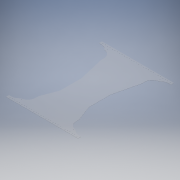
# Autodesk Inventor part: Belly Pan
Saved by Autodesk Inventor 2019.4 (Build 234330000, 330)
## iProperties
Created: 2019-12-14
Part Number: Belly Pan
Material: Polycarbonate, Clear
Document SubType Name: Modeling
Designer: Mark
Density: 1.2 g/cm^3
Appearance: Polycarbonate - Clear
Mass: 741.672 g
Surface Area: 6247.34 cm^2
Volume: 618.06 cm^3
Author: Mark
Autodesk Inventor part; units mm, degrees
ref_plane "YZ Plane" through (0, 0, 0) normal (1, 0, 0) x (0, 1, 0)
ref_plane "XZ Plane" through (0, 0, 0) normal (0, 1, 0) x (-1, 0, 0)
ref_plane "XY Plane" through (0, 0, 0) normal (0, 0, 1) x (1, 0, 0)
sketch "Sketch1" plane through (0, 0, 0) normal (0, 1, 0) x (-1, 0, 0)
  line L0 (-230, 400) -> (230, 400)
  line L1 (230, 400) -> (230, -400)
  line L2 (230, -400) -> (-230, -400)
  line L3 (-230, -400) -> (-230, 400)
  line L4 (-230, 400) -> (230, -400) construction
  line L5 (230, 400) -> (-230, -400) construction
  line L6 (230, 400) -> (300, 400)
  line L7 (300, 400) -> (300, 375)
  line L8 (300, 375) -> (230, 375)
  line L9 (230, 375) -> (230, 400)
  line L10 (230, -400) -> (300, -400)
  line L11 (300, -400) -> (300, -375)
  line L12 (300, -375) -> (230, -375)
  line L13 (230, -375) -> (230, -400)
  line L14 (-230, -400) -> (-300, -400)
  line L15 (-300, -400) -> (-300, -375)
  line L16 (-300, -375) -> (-230, -375)
  line L17 (-230, -375) -> (-230, -400)
  line L18 (-230, 400) -> (-300, 400)
  line L19 (-300, 400) -> (-300, 375)
  line L20 (-300, 375) -> (-230, 375)
  line L21 (-230, 375) -> (-230, 400)
  line L22 (-230, 217.5) -> (-300, 217.5)
  line L23 (-300, 217.5) -> (-300, 192.5)
  line L24 (-300, 192.5) -> (-230, 192.5)
  line L25 (-230, 192.5) -> (-230, 217.5)
  line L26 (230, 217.5) -> (300, 217.5)
  line L27 (300, 217.5) -> (300, 192.5)
  line L28 (300, 192.5) -> (230, 192.5)
  line L29 (230, 192.5) -> (230, 217.5)
  line L30 (-230, -227.5) -> (-300, -227.5)
  line L31 (-300, -227.5) -> (-300, -202.5)
  line L32 (-300, -202.5) -> (-230, -202.5)
  line L33 (-230, -202.5) -> (-230, -227.5)
  line L34 (-230, -87.5) -> (-300, -87.5)
  line L35 (-300, -87.5) -> (-300, -62.5)
  line L36 (-300, -62.5) -> (-230, -62.5)
  line L37 (-230, -62.5) -> (-230, -87.5)
  line L38 (0, 0) -> (0, -50)
  line L39 (0, 0) -> (50, 0) construction
  line L40 (230, -227.5) -> (300, -227.5)
  line L41 (300, -227.5) -> (300, -202.5)
  line L42 (300, -202.5) -> (230, -202.5)
  line L43 (230, -202.5) -> (230, -227.5)
  line L44 (230, -87.5) -> (300, -87.5)
  line L45 (300, -87.5) -> (300, -62.5)
  line L46 (300, -62.5) -> (230, -62.5)
  line L47 (230, -62.5) -> (230, -87.5)
  dimension "d0" = 460
  dimension "d1" = 800
  dimension "d26" = 70
  dimension "d27" = 25
  dimension "d28" = 70
  dimension "d29" = 25
  dimension "d30" = 70
  dimension "d31" = 25
  dimension "d32" = 70
  dimension "d33" = 70
  dimension "d34" = 25
  dimension "d35" = 182.5
  dimension "d36" = 70
  dimension "d37" = 25
  dimension "d38" = 182.5
  dimension "d39" = 70
  dimension "d40" = 25
  dimension "d41" = 172.5
  dimension "d42" = 70
  dimension "d43" = 25
  dimension "d44" = 312.5
  dimension "d45" = 50
  dimension "d46" = 90
  constraints: 96 end point, 18 parallel, 10 horizontal, 10 perpendicular, 8 symmetric about line, 5 point on line, 2 midpoint, 1 vertical
  measures "d0" distance of L1.end L2.end
  measures "d1" distance of L0.end L1.end
  measures "d26" distance of L7.end L8.end
  measures "d27" distance of L6.end L7.end
  measures "d28" distance of L12.end L11.end
  measures "d29" distance of L11.end L10.end
  measures "d30" distance of L15.end L16.end
  measures "d31" distance of L14.end L15.end
  measures "d32" distance of L20.end L19.end
  measures "d33" distance of L24.end L23.end
  measures "d34" distance of L23.end L22.end
  measures "d35" distance between parallel lines of L18 L22
  measures "d36" distance of L27.end L28.end
  measures "d37" distance of L26.end L27.end
  measures "d38" distance between parallel lines of L26 L6
  measures "d39" distance of L31.end L32.end
  measures "d40" distance of L30.end L31.end
  measures "d41" distance between parallel lines of L2 L30
  measures "d42" distance of L35.end L36.end
  measures "d43" distance of L34.end L35.end
  measures "d44" distance between parallel lines of L2 L34
  measures "d45" distance of L38.start L38.end
  measures "d46" angle of L38 L39
extrude "Extrusion1" add sketch "Sketch1" along normal blind 2 contours L0 L1 L2 L3 | L3 L20 L19 L18 | L6 L7 L8 L1 | L3 L14 L15 L16 | L12 L11 L10 L1
sketch "Sketch2" plane through (0, 2, 0) normal (0, 1, 0) x (1, 0, 0)
  line L0 (-230, 375) -> (-230, -375) projected
  line L1 (-230, -130) -> (-120, -130)
  line L2 (-120, -130) -> (-120, 50)
  line L3 (-120, 50) -> (-230, 50)
  line L4 (-230, 50) -> (-230, -130)
  line L5 (300, 400) -> (-300, 400) projected
  line L6 (230, -130) -> (120, -130)
  line L7 (120, -130) -> (120, 50)
  line L8 (120, 50) -> (230, 50)
  line L9 (230, 50) -> (230, -130)
  line L10 (230, -375) -> (230, 375) projected
  line L11 (-230, -40) -> (230, -40) construction
  line L12 (-230, -40) -> (230, -40) construction
  line L13 (-230, -347.5) -> (-170, -347.5)
  line L14 (-170, -347.5) -> (-170, -262.5)
  line L15 (-170, -262.5) -> (-230, -262.5)
  line L16 (-230, -262.5) -> (-230, -347.5)
  line L17 (-300, -400) -> (300, -400) projected
  line L18 (0, -400) -> (0, -300) construction
  line L19 (0, -400) -> (100, -400) construction
  line L20 (230, -347.5) -> (170, -347.5)
  line L21 (170, -347.5) -> (170, -262.5)
  line L22 (170, -262.5) -> (230, -262.5)
  line L23 (230, -262.5) -> (230, -347.5)
  line L24 (-230, 182.5) -> (-230, 267.5)
  line L25 (-230, 347.5) -> (-170, 347.5)
  line L26 (-170, 347.5) -> (-170, 262.5)
  line L27 (-170, 262.5) -> (-230, 262.5)
  line L28 (-230, 262.5) -> (-230, 347.5)
  line L29 (230, 347.5) -> (170, 347.5)
  line L30 (170, 347.5) -> (170, 262.5)
  line L31 (170, 262.5) -> (230, 262.5)
  line L32 (230, 262.5) -> (230, 347.5)
  line L33 (120, 50) -> (170, 262.5)
  line L34 (120, -130) -> (170, -262.5)
  line L35 (-170, -262.5) -> (-120, -130)
  line L36 (-120, -130) -> (-230, -130)
  line L37 (-230, -262.5) -> (-230, -130)
  line L38 (-230, -262.5) -> (-170, -262.5)
  line L39 (-120, 50) -> (-230, 50)
  line L40 (-230, 50) -> (-230, 262.5)
  line L41 (-230, 262.5) -> (-170, 262.5)
  line L42 (-170, 262.5) -> (-120, 50)
  line L43 (-170, -262.5) -> (-230, -262.5)
  line L44 (-230, -262.5) -> (-230, -130)
  line L45 (-230, -130) -> (-120, -130)
  line L46 (-120, -130) -> (-170, -262.5)
  line L47 (-230, 50) -> (-230, 262.5)
  line L48 (-230, 262.5) -> (-170, 262.5)
  line L49 (-170, 262.5) -> (-120, 50)
  line L50 (-120, 50) -> (-230, 50)
  line L51 (120, 50) -> (230, 50)
  line L52 (230, 262.5) -> (230, 50)
  line L53 (120, 50) -> (170, 262.5)
  line L54 (170, 262.5) -> (230, 262.5)
  line L55 (170, -262.5) -> (120, -130)
  line L56 (120, -130) -> (230, -130)
  line L57 (230, -262.5) -> (170, -262.5)
  line L58 (230, -262.5) -> (230, -130)
  point P0 (0, 0)
  point P1 (-230, 400)
  point P2 (-230, -400)
  point P3 (230, 400)
  point P4 (230, -400)
  point P5 (-230, -192.5)
  point P6 (230, -217.5)
  point P7 (-230, 87.5)
  dimension "d4" = 110
  dimension "d5" = 180
  dimension "d6" = 350
  dimension "d7" = 110
  dimension "d8" = 180
  dimension "d9" = 350
  dimension "d12" = 460
  dimension "d13" = 0
  dimension "d14" = 60
  dimension "d15" = 85
  dimension "d16" = 222.5
  dimension "d17" = 100
  dimension "d18" = 90
  dimension "d19" = 60
  dimension "d20" = 85
  dimension "d21" = 52.5
  dimension "d22" = 60
  dimension "d23" = 85
  dimension "d24" = 52.5
  constraints: 110 end point, 13 collinear, 12 parallel, 11 perpendicular, 7 horizontal, 6 symmetric about line, 3 vertical, 2 equal length, 2 midpoint, 1 point on line, 4 other
  measures "d4" distance of L3.end L2.end
  measures "d5" distance of L2.end L1.end
  measures "d6" distance between parallel lines of L5 L3
  measures "d7" distance of L7.end L8.end
  measures "d8" distance of L6.end L7.end
  measures "d9" distance between parallel lines of L5 L8
  measures "d12" distance of L11.start L11.end
  measures "d13" distance between parallel lines of L12 L11
  measures "d14" distance of L15.end L14.end
  measures "d15" distance of L14.end L13.end
  measures "d16" distance between parallel lines of L11 L15
  measures "d17" distance of L18.start L18.end
  measures "d18" angle of L19 L18
  measures "d19" distance of L26.end L27.end
  measures "d20" distance of L25.end L26.end
  measures "d21" distance between parallel lines of L5 L25
  measures "d22" distance of L31.end L30.end
  measures "d23" distance of L30.end L29.end
  measures "d24" distance between parallel lines of L5 L29
extrude "Extrusion2" cut sketch "Sketch2" against normal blind 3
fillet "Fillet1" radius 60 20 edges at (120, 1, 130) (120, 1, -50) (170, 1, 262.5) (170, 1, 347.5) (170, 1, -262.5) (170, 1, -347.5) (-170, 1, 347.5) (-170, 1, 262.5) (-120, 1, 130) (-120, 1, -50) (-170, 1, -262.5) (-170, 1, -347.5) (230, 1, 375) (230, 1, 347.5) (-230, 1, 347.5) (-230, 1, 375) (-230, 1, -347.5) (-230, 1, -375) (230, 1, -375) (230, 1, -347.5)
sketch "Sketch3" plane through (0, 2, 0) normal (0, 1, 0) x (1, 0, 0)
  circle A0 centre (-217.5, 345) radius 2.75 projected
  circle A1 centre (-217.5, 305) radius 2.75 projected
  circle A2 centre (-217.5, 265) radius 2.75 projected
  circle A3 centre (-217.5, 225) radius 2.75 projected
  circle A4 centre (-217.5, 185) radius 2.75 projected
  circle A5 centre (-217.5, 145) radius 2.75 projected
  circle A6 centre (-217.5, 105) radius 2.75 projected
  circle A7 centre (-217.5, 65) radius 2.75 projected
  circle A8 centre (-217.5, 25) radius 2.75 projected
  circle A9 centre (-217.5, -15) radius 2.75 projected
  circle A10 centre (-217.5, -55) radius 2.75 projected
  circle A11 centre (-217.5, -95) radius 2.75 projected
  circle A12 centre (-217.5, -135) radius 2.75 projected
  circle A13 centre (-217.5, -175) radius 2.75 projected
  circle A14 centre (-217.5, -215) radius 2.75 projected
  circle A15 centre (-217.5, -255) radius 2.75 projected
  circle A16 centre (-217.5, -295) radius 2.75 projected
  circle A17 centre (-217.5, -335) radius 2.75 projected
  circle A18 centre (-217.5, -355) radius 2.75 projected
  circle A19 centre (-217.5, -315) radius 2.75 projected
  circle A20 centre (-217.5, -275) radius 2.75 projected
  circle A21 centre (-217.5, -235) radius 2.75 projected
  circle A22 centre (-217.5, -195) radius 2.75 projected
  circle A23 centre (-217.5, -155) radius 2.75 projected
  circle A24 centre (-217.5, -115) radius 2.75 projected
  circle A25 centre (-217.5, -75) radius 2.75 projected
  circle A26 centre (-217.5, -35) radius 2.75 projected
  circle A27 centre (-217.5, 5) radius 2.75 projected
  circle A28 centre (-217.5, 45) radius 2.75 projected
  circle A29 centre (-217.5, 85) radius 2.75 projected
  circle A30 centre (-217.5, 125) radius 2.75 projected
  circle A31 centre (-217.5, 165) radius 2.75 projected
  circle A32 centre (-217.5, 205) radius 2.75 projected
  circle A33 centre (-217.5, 245) radius 2.75 projected
  circle A34 centre (-217.5, 285) radius 2.75 projected
  circle A35 centre (-217.5, 325) radius 2.75 projected
  circle A36 centre (-217.5, 365) radius 2.75 projected
  line L0 (-205, -375) -> (-230, -375) projected
  line L1 (-205, -375) -> (-205, 375) projected
  line L2 (-205, 375) -> (-230, 375) projected
  line L3 (-230, -375) -> (-230, 375) projected
  circle A37 centre (-245, -205) radius 2.75 projected
  circle A38 centre (-265, -205) radius 2.75 projected
  circle A39 centre (-285, -205) radius 2.75 projected
  circle A40 centre (-280, -387.5) radius 2.75 projected
  circle A41 centre (-260, -387.5) radius 2.75 projected
  circle A42 centre (-220, -387.5) radius 2.75 projected
  circle A43 centre (-180, -387.5) radius 2.75 projected
  circle A44 centre (-140, -387.5) radius 2.75 projected
  circle A45 centre (-100, -387.5) radius 2.75 projected
  circle A46 centre (-60, -387.5) radius 2.75 projected
  circle A47 centre (-20, -387.5) radius 2.75 projected
  circle A48 centre (20, -387.5) radius 2.75 projected
  circle A49 centre (60, -387.5) radius 2.75 projected
  circle A50 centre (100, -387.5) radius 2.75 projected
  circle A51 centre (140, -387.5) radius 2.75 projected
  circle A52 centre (180, -387.5) radius 2.75 projected
  circle A53 centre (220, -387.5) radius 2.75 projected
  circle A54 centre (260, -387.5) radius 2.75 projected
  circle A55 centre (280, -387.5) radius 2.75 projected
  circle A56 centre (240, -387.5) radius 2.75 projected
  circle A57 centre (200, -387.5) radius 2.75 projected
  circle A58 centre (160, -387.5) radius 2.75 projected
  circle A59 centre (120, -387.5) radius 2.75 projected
  circle A60 centre (80, -387.5) radius 2.75 projected
  circle A61 centre (40, -387.5) radius 2.75 projected
  circle A62 centre (0, -387.5) radius 2.75 projected
  circle A63 centre (-40, -387.5) radius 2.75 projected
  circle A64 centre (-80, -387.5) radius 2.75 projected
  circle A65 centre (-120, -387.5) radius 2.75 projected
  circle A66 centre (-160, -387.5) radius 2.75 projected
  circle A67 centre (-200, -387.5) radius 2.75 projected
  circle A68 centre (-240, -387.5) radius 2.75 projected
  circle A69 centre (-280, -387.5) radius 2.75 projected
  line L4 (300, -397) -> (300, -378) projected
  line L5 (300, -397) -> (-300, -397) projected
  line L6 (-300, -378) -> (-300, -397) projected
  line L7 (300, -378) -> (-300, -378) projected
  circle A70 centre (-265, 75) radius 2.75 projected
  circle A71 centre (-245, 75) radius 2.75 projected
  circle A72 centre (-285, 75) radius 2.75 projected
  line L8 (-230, 87.5) -> (-230, 62.5) projected
  line L9 (-230, 62.5) -> (-300, 62.5) projected
  line L10 (-300, 62.5) -> (-300, 87.5) projected
  line L11 (-230, 87.5) -> (-300, 87.5) projected
  circle A73 centre (-265, -205) radius 2.75 projected
  circle A74 centre (-245, -205) radius 2.75 projected
  circle A75 centre (-285, -205) radius 2.75 projected
  line L12 (-230, -192.5) -> (-230, -217.5) projected
  line L13 (-230, -217.5) -> (-300, -217.5) projected
  line L14 (-300, -217.5) -> (-300, -192.5) projected
  line L15 (-230, -192.5) -> (-300, -192.5) projected
  circle A76 centre (-265, 215) radius 2.75 projected
  circle A77 centre (-245, 215) radius 2.75 projected
  circle A78 centre (-285, 215) radius 2.75 projected
  line L16 (-230, 227.5) -> (-230, 202.5) projected
  line L17 (-230, 202.5) -> (-300, 202.5) projected
  line L18 (-300, 202.5) -> (-300, 227.5) projected
  line L19 (-230, 227.5) -> (-300, 227.5) projected
  circle A79 centre (260, 387.5) radius 2.75 projected
  circle A80 centre (220, 387.5) radius 2.75 projected
  circle A81 centre (180, 387.5) radius 2.75 projected
  circle A82 centre (140, 387.5) radius 2.75 projected
  circle A83 centre (100, 387.5) radius 2.75 projected
  circle A84 centre (60, 387.5) radius 2.75 projected
  circle A85 centre (20, 387.5) radius 2.75 projected
  circle A86 centre (-20, 387.5) radius 2.75 projected
  circle A87 centre (-60, 387.5) radius 2.75 projected
  circle A88 centre (-100, 387.5) radius 2.75 projected
  circle A89 centre (-140, 387.5) radius 2.75 projected
  circle A90 centre (-180, 387.5) radius 2.75 projected
  circle A91 centre (-220, 387.5) radius 2.75 projected
  circle A92 centre (-260, 387.5) radius 2.75 projected
  circle A93 centre (-280, 387.5) radius 2.75 projected
  circle A94 centre (-240, 387.5) radius 2.75 projected
  circle A95 centre (-200, 387.5) radius 2.75 projected
  circle A96 centre (-160, 387.5) radius 2.75 projected
  circle A97 centre (-120, 387.5) radius 2.75 projected
  circle A98 centre (-80, 387.5) radius 2.75 projected
  circle A99 centre (-40, 387.5) radius 2.75 projected
  circle A100 centre (0, 387.5) radius 2.75 projected
  circle A101 centre (40, 387.5) radius 2.75 projected
  circle A102 centre (80, 387.5) radius 2.75 projected
  circle A103 centre (120, 387.5) radius 2.75 projected
  circle A104 centre (160, 387.5) radius 2.75 projected
  circle A105 centre (200, 387.5) radius 2.75 projected
  circle A106 centre (240, 387.5) radius 2.75 projected
  circle A107 centre (280, 387.5) radius 2.75 projected
  line L20 (-300, 397) -> (-300, 378) projected
  line L21 (-300, 397) -> (300, 397) projected
  line L22 (300, 378) -> (300, 397) projected
  line L23 (-300, 378) -> (300, 378) projected
  circle A108 centre (217.5, 345) radius 2.75 projected
  circle A109 centre (217.5, 305) radius 2.75 projected
  circle A110 centre (217.5, 265) radius 2.75 projected
  circle A111 centre (217.5, 225) radius 2.75 projected
  circle A112 centre (217.5, 185) radius 2.75 projected
  circle A113 centre (217.5, 145) radius 2.75 projected
  circle A114 centre (217.5, 105) radius 2.75 projected
  circle A115 centre (217.5, 65) radius 2.75 projected
  circle A116 centre (217.5, 25) radius 2.75 projected
  circle A117 centre (217.5, -15) radius 2.75 projected
  circle A118 centre (217.5, -55) radius 2.75 projected
  circle A119 centre (217.5, -95) radius 2.75 projected
  circle A120 centre (217.5, -135) radius 2.75 projected
  circle A121 centre (217.5, -175) radius 2.75 projected
  circle A122 centre (217.5, -215) radius 2.75 projected
  circle A123 centre (217.5, -255) radius 2.75 projected
  circle A124 centre (217.5, -295) radius 2.75 projected
  circle A125 centre (217.5, -335) radius 2.75 projected
  circle A126 centre (217.5, -355) radius 2.75 projected
  circle A127 centre (217.5, -315) radius 2.75 projected
  circle A128 centre (217.5, -275) radius 2.75 projected
  circle A129 centre (217.5, -235) radius 2.75 projected
  circle A130 centre (217.5, -195) radius 2.75 projected
  circle A131 centre (217.5, -155) radius 2.75 projected
  circle A132 centre (217.5, -115) radius 2.75 projected
  circle A133 centre (217.5, -75) radius 2.75 projected
  circle A134 centre (217.5, -35) radius 2.75 projected
  circle A135 centre (217.5, 5) radius 2.75 projected
  circle A136 centre (217.5, 45) radius 2.75 projected
  circle A137 centre (217.5, 85) radius 2.75 projected
  circle A138 centre (217.5, 125) radius 2.75 projected
  circle A139 centre (217.5, 165) radius 2.75 projected
  circle A140 centre (217.5, 205) radius 2.75 projected
  circle A141 centre (217.5, 245) radius 2.75 projected
  circle A142 centre (217.5, 285) radius 2.75 projected
  circle A143 centre (217.5, 325) radius 2.75 projected
  circle A144 centre (217.5, 365) radius 2.75 projected
  line L24 (230, -375) -> (205, -375) projected
  line L25 (205, -375) -> (205, 375) projected
  line L26 (230, 375) -> (205, 375) projected
  line L27 (230, -375) -> (230, 375) projected
  circle A145 centre (265, 215) radius 2.75 projected
  circle A146 centre (245, 215) radius 2.75 projected
  circle A147 centre (285, 215) radius 2.75 projected
  line L28 (230, 227.5) -> (230, 202.5) projected
  line L29 (230, 227.5) -> (300, 227.5) projected
  line L30 (300, 202.5) -> (300, 227.5) projected
  line L31 (230, 202.5) -> (300, 202.5) projected
  circle A148 centre (265, 75) radius 2.75 projected
  circle A149 centre (245, 75) radius 2.75 projected
  circle A150 centre (285, 75) radius 2.75 projected
  line L32 (230, 87.5) -> (230, 62.5) projected
  line L33 (230, 87.5) -> (300, 87.5) projected
  line L34 (300, 62.5) -> (300, 87.5) projected
  line L35 (230, 62.5) -> (300, 62.5) projected
  circle A151 centre (265, -205) radius 2.75 projected
  circle A152 centre (245, -205) radius 2.75 projected
  circle A153 centre (285, -205) radius 2.75 projected
  line L36 (230, -192.5) -> (230, -217.5) projected
  line L37 (230, -192.5) -> (300, -192.5) projected
  line L38 (300, -217.5) -> (300, -192.5) projected
  line L39 (230, -217.5) -> (300, -217.5) projected
  point P0 (0, 0)
extrude "Extrusion3" cut sketch "Sketch3" against normal blind 10 contours A0 | A1 | A2 | A3 | A4 | A5 | A6 | A7 | A8 | A9 | A10 | A11 | A12 | A13 | A14 | A15 | A16 | A17 | A18 | A19 | A20 | A21 | A22 | A23 | A24 | A25 | A26 | A27 | A28 | A29 | A30 | A31 | A32 | A33 | A34 | A35 | A36 | A37 | A38 | A39 | A40 | A41 | A42 | A43 | A44 | A45 | A46 | A47 | A48 | A49 | A50 | A51 | A52 | A53 | A54 | A55 | A56 | A57 | A58 | A59 | A60 | A61 | A62 | A63 | A64 | A65 | A66 | A67 | A68 | A70 | A71 | A72 | A76 | A77 | A78 | A79 | A80 | A81 | A82 | A83 | A84 | A85 | A86 | A87 | A88 | A89 | A90 | A91 | A92 | A93 | A94 | A95 | A96 | A97 | A98 | A99 | A100 | A101 | A102 | A103 | A104 | A105 | A106 | A107 | A108 | A109 | A110 | A111 | A112 | A113 | A114 | A115 | A116 | A117 | A118 | A119 | A120 | A121 | A122 | A123 | A124 | A125 | A126 | A127 | A128 | A129 | A130 | A131 | A132 | A133 | A134 | A135 | A136 | A137 | A138 | A139 | A140 | A141 | A142 | A143 | A144 | A145 | A146 | A147 | A148 | A149 | A150 | A151 | A152 | A153
body "Solid1"
